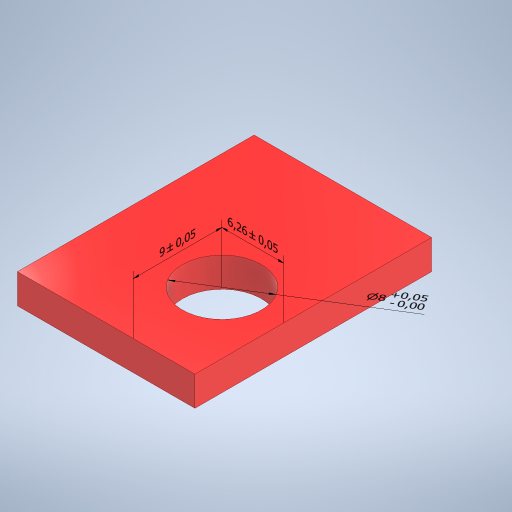
# Autodesk Inventor part: rapoukLegBasev3
Saved by Autodesk Inventor 2024 (Build 280153000, 153)
## iProperties
Created: 2023-10-12
Part Number: rapoukLegBasev3
Material: EN AW-6060 T6
Document SubType Name: Modeling
Designer: Roman Suk
Density: 2.7 g/cm^3
Appearance: Light Red
Author: Roman Suk
Autodesk Inventor part; units mm, degrees
ref_plane "YZ Plane" through (0, 0, 0) normal (1, 0, 0) x (0, 1, 0)
ref_plane "XZ Plane" through (0, 0, 0) normal (0, 1, 0) x (-1, 0, 0)
ref_plane "XY Plane" through (0, 0, 0) normal (0, 0, 1) x (1, 0, 0)
sketch "Sketch1" plane through (0, 0, 0) normal (0, 1, 0) x (-1, 0, 0)
  line L0 (-9, 12) -> (9, 12)
  line L1 (9, 12) -> (9, -12)
  line L2 (9, -12) -> (-9, -12)
  line L3 (-9, -12) -> (-9, 12)
  line L4 (-9, 12) -> (9, -12) construction
  line L5 (9, 12) -> (-9, -12) construction
  circle A0 centre (-2.74, 3) radius 4
  point P0 (0, 0)
  dimension "d0" = 18
  dimension "d1" = 24
  dimension "d2" = 8
  dimension "d3" = 9
  dimension "d9" = 6.26
  constraints: 12 end point, 2 midpoint, 2 parallel, 1 centre point, 1 horizontal, 1 perpendicular
  measures "d0" distance of L1.end L2.end
  measures "d1" distance of L0.end L1.end
  measures "d2" diameter of A0
  measures "d3" distance from line of A0.centre L0
  measures "d9" distance from line of L3 A0.centre
extrude "Extrusion1" add sketch "Sketch1" along normal blind 3
body "Solid1"
